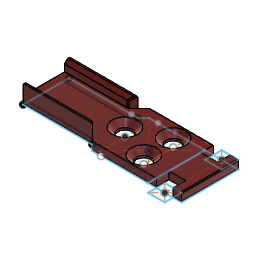
Formbot noname chain FIX v1 (Autodesk Fusion 360 design; units mm, degrees)
Autodesk Fusion 360 part; units mm, degrees
sketch "Sketch1" plane through (0, 0, 0) normal (0, 0, 1) x (1, 0, 0)
  line L0 (6.65, -6.8) -> (-6.65, -6.8)
  line L1 (-6.65, 6.8) -> (6.65, 6.8)
  line L2 (6.65, 6.8) -> (6.65, -6.8)
  line L3 (6.65, -6.8) -> (-6.65, 6.8) construction
  line L4 (-6.65, -6.8) -> (6.65, 6.8) construction
  line L5 (-6.65, 6.8) -> (-7.9935, 5.4565)
  line L6 (-6.65, 6.8) -> (-4.5501, 6.8) construction
  line L7 (-6.65, -6.8) -> (-7.9935, -5.4565)
  line L8 (-6.65, -6.8) -> (-4.5501, -6.8) construction
  line L9 (-7.9935, 5.4565) -> (-24.4935, 5.4565)
  line L10 (-7.9935, -5.4565) -> (-24.4935, -5.4565)
  line L11 (-24.4935, -5.4565) -> (-24.4935, 5.4565)
  line L12 (-5.65, 6.8) -> (-5.65, -6.8) construction
  line L13 (2.35, 6.8) -> (2.35, -6.8) construction
  line L14 (2.35, 0) -> (2.35, 3.5) construction
  line L15 (2.35, 0) -> (2.35, -3.5) construction
  line L16 (6.65, 6.8) -> (14.65, 6.8)
  line L17 (14.65, 6.8) -> (14.65, -6.8)
  line L18 (14.65, -6.8) -> (6.65, -6.8)
  line L19 (6.65, -6.8) -> (6.65, 6.8)
  line L20 (10.65, 6.8) -> (10.65, -6.8) construction
  line L21 (12.65, 4.8) -> (8.65, 4.8)
  line L22 (8.65, 4.8) -> (8.65, 8.8)
  line L23 (8.65, 8.8) -> (12.65, 8.8)
  line L24 (12.65, 8.8) -> (12.65, 4.8)
  line L25 (12.65, 4.8) -> (8.65, 8.8) construction
  line L26 (8.65, 4.8) -> (12.65, 8.8) construction
  line L27 (12.65, -8.8) -> (8.65, -8.8)
  line L28 (8.65, -8.8) -> (8.65, -4.8)
  line L29 (8.65, -4.8) -> (12.65, -4.8)
  line L30 (12.65, -4.8) -> (12.65, -8.8)
  line L31 (12.65, -8.8) -> (8.65, -4.8) construction
  line L32 (8.65, -8.8) -> (12.65, -4.8) construction
  point P0 (-5.65, 0)
  point P1 (10.65, 6.8)
  point P2 (10.65, -6.8)
  dimension "d1" = 13.3
  dimension "d2" = 13.6
  dimension "d3" = 135
  dimension "d4" = 1.9
  dimension "d5" = 135
  dimension "d6" = 1.9
  dimension "d7" = 16.5
  dimension "d8" = 12.3
  dimension "d9" = 4.3
  dimension "d10" = 3.5
  dimension "d11" = 3.5
  dimension "d19" = 8
  dimension "d20" = 4
  dimension "d21" = 4
  dimension "d22" = 4
  dimension "d23" = 4
  constraint horizontal L0
  constraint parallel L0 L1
  constraint coincident L3 origin
  constraint coincident L4 origin
  constraint horizontal L6
  constraint horizontal L8
  constraint perpendicular L9 L11
  constraint coincident L1 L12.start
  constraint coincident L0 L12.end
  constraint perpendicular L0 L12
  constraint midpoint L12 P0
  constraint coincident L1 L13.start
  constraint coincident L0 L13.end
  constraint perpendicular L0 L13
  constraint midpoint L13 L14.start
  constraint parallel L13 L14
  constraint parallel L13 L15
  constraint horizontal L16
  constraint vertical L17
  constraint horizontal L18
  constraint vertical L19
  constraint midpoint L16 P1
  constraint midpoint L18 P2
  constraint horizontal L21
  constraint perpendicular L21 L22
  constraint parallel L21 L23
  constraint parallel L22 L24
  constraint coincident L25 P1
  constraint coincident L26 P1
  constraint coincident P1 L20.start
  constraint horizontal L27
  constraint perpendicular L27 L28
  constraint parallel L27 L29
  constraint parallel L28 L30
  constraint coincident L31 P2
  constraint coincident L32 P2
  constraint coincident P2 L20.end
  measures "d1" distance of L1.start L1.end
  measures "d2" distance of L0.end L1.start
  measures "d3" angle of L5 L6
  measures "d4" distance of L1.start L5.end
  measures "d5" angle of L7 L8
  measures "d6" distance of L0.end L7.end
  measures "d7" distance of L5.end L9.end
  measures "d8" distance of L2 L12
  measures "d9" distance of L2 L13
  measures "d10" distance of L14.start L14.end
  measures "d11" distance of L14.start L15.end
  measures "d19" distance of L1.end L16.end
  measures "d20" distance of L22.end L23.end
  measures "d21" distance of L21.end L22.end
  measures "d22" distance of L28.end L29.end
  measures "d23" distance of L27.end L28.end
extrude "Extrude1" add sketch "Sketch1" against normal blind 1.8 contours L0 L1 L2 L5 L7 L9 L10 L11 L19
hole "Hole1" at (2.35, 3.5, 0) at (2.35, -3.5, 0) at (-5.65, 0, 0) direction (0, 0, -1) diameter 3.4 depth 4231.15 tip angle 180 countersink diameter 6 countersink angle 90
extrude "Extrude2" add sketch "Sketch1" against normal up to surface (1.8 mm away) contours L2 L16 L17 L18 L19 L21 L22 L24 L28 L29 L30
sketch "Sketch2" plane through (0, 0, 0) normal (0, 0, 1) x (-1, 0, 0)
  circle A0 centre (-2.35, 3.5) radius 3
  circle A1 centre (-2.35, -3.5) radius 3
  circle A2 centre (5.65, 0) radius 3
  line L0 (6.65, -6.8) -> (7.9935, -5.4565)
  line L1 (7.9935, -5.4565) -> (24.4935, -5.4565)
  line L2 (24.4935, -5.4565) -> (24.4935, 5.4565)
  line L3 (24.4935, 5.4565) -> (7.9935, 5.4565)
  line L4 (7.9935, 5.4565) -> (6.65, 6.8)
  line L5 (6.65, 6.8) -> (-8.65, 6.8)
  line L6 (-8.65, 6.8) -> (-8.65, 4.8)
  line L7 (-8.65, 4.8) -> (-12.65, 4.8)
  line L8 (-12.65, 4.8) -> (-12.65, 6.8)
  line L9 (-12.65, 6.8) -> (-14.65, 6.8)
  line L10 (-14.65, 6.8) -> (-14.65, -6.8)
  line L11 (-14.65, -6.8) -> (-12.65, -6.8)
  line L12 (-12.65, -6.8) -> (-12.65, -4.8)
  line L13 (-12.65, -4.8) -> (-8.65, -4.8)
  line L14 (-8.65, -4.8) -> (-8.65, -6.8)
  line L15 (-8.65, -6.8) -> (6.65, -6.8)
  line L16 (24.4935, -5.4565) -> (24.4935, -4.2565)
  line L17 (7.9935, -5.4565) -> (9.1935, -4.2565)
  line L18 (7.9935, -5.4565) -> (9.5491, -5.4565) construction
  line L19 (24.4935, 5.4565) -> (24.4935, 4.2565) construction
  line L20 (7.9935, 5.4565) -> (9.1935, 4.2565)
  line L21 (24.4935, -4.2565) -> (9.1935, -4.2565)
  line L22 (24.4935, 4.2565) -> (9.1935, 4.2565)
  dimension "d26" = 1.2
  dimension "d27" = 45
  dimension "d28" = 1.2
  constraint coincident L1.end L2.start
  constraint perpendicular L1 L16
  constraint horizontal L18
  constraint coincident L0.end L1.start
  constraint coincident L2.end L3.start
  constraint perpendicular L3 L19
  constraint coincident L3.end L4.start
  constraint parallel L4 L20
  constraint perpendicular L16 L21
  constraint perpendicular L19 L22
  measures "d26" distance of L1.end L16.end
  measures "d27" angle of L17 L18
  measures "d28" distance of L2.end L19.end
extrude "Extrude3" add sketch "Sketch2" along normal blind 2.4 contours L1 L2 L16 L17 L21 | L2 L3 L20 L22
chamfer "Chamfer1" distance 0.8 angle 45 2 edges at (-16.8435, 4.2565, 2.4) (-16.8435, -4.2565, 2.4)
chamfer "Chamfer2" distance 0.2 angle 45 14 edges at (14.65, 0, 0) (-24.4935, 0, 0) (-24.4935, 4.2565, 0.8) (-24.4935, 4.6565, 2) (-24.4935, 5.2565, 2.4) (-24.4935, -4.2565, 0.8) (-24.4935, -4.6565, 2) (-24.4935, -5.2565, 2.4) (-8.1935, 5.2565, 2.4) (-8.7935, 4.6565, 2) (-9.1935, 4.2565, 0.8) (-9.1935, -4.2565, 0.8) (-8.7935, -4.6565, 2) (-8.1935, -5.2565, 2.4)
move_body "Move1" bodies 1 to x (1, 0, 0) y (0, 1, 0) z (0, 0, 1) at (0, 0, 2)
extrude "Extrude4" cut 1 faces at (9.9833, -4.8, 1.4) along direction (0, 1, 0) blind 1
extrude "Extrude5" cut 1 faces at (11.3167, 4.8, 1.4) along direction (0, -1, 0) blind 1
named bodies: "Formbot-chain-fix-10x11"
